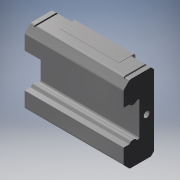
# Autodesk Inventor part: SRS12MSS Slider
Saved by Autodesk Inventor 2016 (Build 200138000, 138)
## iProperties
Category: PARTsolutions
Company: THK
Created: 2015-05-12
Part Number: SRS12MSS Slider
Catalog Web Link: www.cadenas.de
Description: Compact Type SRS-M Slider-
Vendor: THK
Document SubType Name: Modeling
Designer: PARTuser1
Manufacturer: THK
Mass: 57.6277 g
Surface Area: 35.5033 cm^2
Volume: 7.45507 cm^3
Density: 7.73 g/cm^3
Material: Steel, Alloy
Appearance: Semi-Polished
PSOL_IDENT_0: {$CADENAS_DATA\23d-libs\thk\linear_motion_systems\lm_guide\lm_caged_ball_roller\caged_ball\lm_guide_
PSOL_IDENT_1: srs\srs_m\srs_m_slider.prj},201 {VTYP=3D},{NB=SRS12MSS Slider},{LINA=SRS12MSS Slider},{NN=Compact Ty
PSOL_IDENT_2: pe SRS-M Slider},{DATE=07.01.2015 08:42:03},{GEOMDATE=07.01.2015 08:42:03},{VERSION=},{LINEID=130},{
PSOL_IDENT_3: LINESUBID=-1},{WBVAR=QZ,SO,GPJ}  {NB=SRS12MSS Slider},{LINA=SRS12MSS Slider},{KT=DUMMY},{MN=SRS12M},
PSOL_IDENT_4: {ND=3.000},{QZ=},{SO=SS},{SO1='SS','SS- With end seals, side seals','UU','UU- With end seals (on bot
PSOL_IDENT_5: h ends)','SSHH','SSHH- With end seals, side seals and LaCS'},{GPJ=},{M=13.00},{W=27.00},{K=11.00},{L=
PSOL_IDENT_6: 34.40},{L1=20.60},{LX=34.4},{B=20.00},{C=15.00},{S=3.00},{SL=3.200},{T=5.70},{N=3.00},{GPJ1='', 'Non
PSOL_IDENT_7: e'},{L4=0},{V=3.250},{M1=7.500},{X=3.500},{Y=2.000},{X1=0.500},{X2=26.800},{X3=4.800},{X4=3.000},{X5=
PSOL_IDENT_8: 3.000},{W1=12.000},{L3=5.400},{H3=2.000},{H=0.000},{QZ1='', 'No', 'QZ', 'Yes'},{UD1=21.000},{UD2=8.0
PSOL_IDENT_9: 00},{R=1.800},{VER=2},{VER2=2}
SUPPLIER: THK
ARTICLENO: SRS12MSS Slider
BOMINFO: SRS12MSS Slider
CREATOR: CADENAS GmbH
Title: SRS12MSS Slider
Author: Cadenas PARTsolutions
Autodesk Inventor part; units mm, degrees
sketch "Sketch_3" plane through (0, 0, 0) normal (1, 0, 0) x (0, 1, 0)
  line L0 (10.5, 13.5) -> (5.3, 13.5)
  line L1 (5.3, 13.5) -> (5.24, 13.4)
  line L2 (5.24, 13.4) -> (2.5142, 13.4)
  arc A0 (2.5142, 13.4) -> (1.8071, 13.1071) centre (2.5142, 12.4) ccw
  line L3 (1.8071, 13.1071) -> (0.2929, 11.5929)
  arc A1 (0.2929, 11.5929) -> (0, 10.8858) centre (1, 10.8858) ccw
  line L4 (0, 10.8858) -> (0, -10.8858)
  arc A2 (0, -10.8858) -> (0.2929, -11.5929) centre (1, -10.8858) ccw
  line L5 (0.2929, -11.5929) -> (1.8071, -13.1071)
  arc A3 (1.8071, -13.1071) -> (2.5142, -13.4) centre (2.5142, -12.4) ccw
  line L6 (2.5142, -13.4) -> (5.24, -13.4)
  line L7 (5.24, -13.4) -> (5.3, -13.5)
  line L8 (5.3, -13.5) -> (10.5, -13.5)
  line L9 (10.5, -13.5) -> (11, -13)
  line L10 (11, -13) -> (11, -6)
  line L11 (11, -6) -> (10.7713, -5.6188)
  arc A4 (10.7, -5.3615) -> (10.7713, -5.6188) centre (11.2, -5.3615) ccw
  line L12 (10.7, -5.3615) -> (10.7, 5.3615)
  arc A5 (10.7713, 5.6188) -> (10.7, 5.3615) centre (11.2, 5.3615) ccw
  line L13 (10.7713, 5.6188) -> (11, 6)
  line L14 (11, 6) -> (11, 13)
  line L15 (11, 13) -> (10.5, 13.5)
  constraints: 32 end point, 12 point on circle, 6 centre point
extrude "Extrusion1" add sketch "Sketch_3" along normal mid plane 20.6
sketch "Sketch_9" plane through (10.3, 0, 0) normal (1, 0, 0) x (0, 0, -1)
  arc A0 (-13.4, 2.5142) -> (-13.1071, 1.8071) centre (-12.4, 2.5142) ccw
  line L0 (-13.1071, 1.8071) -> (-11.5929, 0.2929)
  arc A1 (-11.5929, 0.2929) -> (-10.8858, 0) centre (-10.8858, 1) ccw
  line L1 (-10.8858, 0) -> (10.8858, 0)
  arc A2 (10.8858, 0) -> (11.5929, 0.2929) centre (10.8858, 1) ccw
  line L2 (11.5929, 0.2929) -> (13.1071, 1.8071)
  arc A3 (13.1071, 1.8071) -> (13.4, 2.5142) centre (12.4, 2.5142) ccw
  line L3 (13.4, 2.5142) -> (13.4, 9.5)
  line L4 (13.4, 9.5) -> (12.4, 10.5)
  line L5 (12.4, 10.5) -> (-12.4, 10.5)
  line L6 (-12.4, 10.5) -> (-13.4, 9.5)
  line L7 (-13.4, 9.5) -> (-13.4, 2.5142)
  constraints: 16 end point, 8 point on circle, 4 centre point
extrude "Extrusion2" add sketch "Sketch_9" along normal blind 6.9
sketch "Sketch_15" plane through (-10.3, 0, 0) normal (1, 0, 0) x (0, 0, -1)
  arc A0 (-13.4, 2.5142) -> (-13.1071, 1.8071) centre (-12.4, 2.5142) ccw
  line L0 (-13.1071, 1.8071) -> (-11.5929, 0.2929)
  arc A1 (-11.5929, 0.2929) -> (-10.8858, 0) centre (-10.8858, 1) ccw
  line L1 (-10.8858, 0) -> (10.8858, 0)
  arc A2 (10.8858, 0) -> (11.5929, 0.2929) centre (10.8858, 1) ccw
  line L2 (11.5929, 0.2929) -> (13.1071, 1.8071)
  arc A3 (13.1071, 1.8071) -> (13.4, 2.5142) centre (12.4, 2.5142) ccw
  line L3 (13.4, 2.5142) -> (13.4, 9.5)
  line L4 (13.4, 9.5) -> (12.4, 10.5)
  line L5 (12.4, 10.5) -> (-12.4, 10.5)
  line L6 (-12.4, 10.5) -> (-13.4, 9.5)
  line L7 (-13.4, 9.5) -> (-13.4, 2.5142)
  constraints: 16 end point, 8 point on circle, 4 centre point
extrude "Extrusion3" add sketch "Sketch_15" against normal blind 6.9
sketch "Sketch_40" plane through (0, 0, 0) normal (1, 0, 0) x (0, 1, 0)
  line L0 (-1.5, 6) -> (-2, 5.5)
  line L1 (-2, 5.5) -> (-2, -5.5)
  line L2 (-2, -5.5) -> (-1.5, -6)
  line L3 (-1.5, -6) -> (1.9874, -6)
  arc A0 (3.3, -5.2629) -> (1.9874, -6) centre (3.21, -6.64) ccw
  arc A1 (4.6126, -6) -> (3.3, -5.2629) centre (3.39, -6.64) ccw
  line L4 (4.6126, -6) -> (5.2, -6)
  line L5 (5.2, -6) -> (5.5, -5.7)
  line L6 (5.5, -5.7) -> (5.5, 5.7)
  line L7 (5.5, 5.7) -> (5.2, 6)
  line L8 (5.2, 6) -> (4.6126, 6)
  arc A2 (3.3, 5.2629) -> (4.6126, 6) centre (3.39, 6.64) ccw
  arc A3 (1.9874, 6) -> (3.3, 5.2629) centre (3.21, 6.64) ccw
  line L9 (1.9874, 6) -> (-1.5, 6)
  constraints: 20 end point, 8 point on circle, 4 centre point
extrude "Extrusion4" cut sketch "Sketch_40" along normal mid plane 34.4
sketch "Sketch5" plane through (-10.3, 11, 6) normal (0, 1, 0) x (1, 0, 0)
  point P0 (17.8, -4)
hole "Hole1" at (7.5, 11, 10) direction (0, -1, 0) diameter 2.459 depth 3.84 tip angle 120 countersink diameter 3 countersink angle 90 thread size "M3x0.5" class "6H" standard "ISO Metric profile"
pattern_linear "Rectangular Pattern1" count 2 spacing 20 along (0, 0, -1) count 2 spacing 15 along (-1, 0, 0) of "Hole1"
sketch "Sketch_38" plane through (0, 0, 0) normal (0, 0, 1) x (1, 0, 0)
  line L0 (15.2, 10.5) -> (15.7, 10)
  line L1 (15.7, 10) -> (15.7, 10.5)
  line L2 (15.7, 10.5) -> (15.2, 10.5)
  constraints: 6 end point
extrude "Extrusion5" cut sketch "Sketch_38" along normal mid plane 26.8
sketch "Sketch_39" plane through (0, 0, 0) normal (0, 0, 1) x (1, 0, 0)
  line L0 (-15.7, 10.5) -> (-15.7, 10)
  line L1 (-15.7, 10) -> (-15.2, 10.5)
  line L2 (-15.2, 10.5) -> (-15.7, 10.5)
  constraints: 6 end point
extrude "Extrusion6" cut sketch "Sketch_39" along normal mid plane 26.8
sketch "Sketch_21" plane through (0, 0, 0) normal (0, 1, 0) x (-1, 0, 0)
  line L0 (15.7, -13.4) -> (15.7, -12.9)
  line L1 (15.7, -12.9) -> (15.2, -13.4)
  line L2 (15.2, -13.4) -> (15.7, -13.4)
  constraints: 6 end point
extrude "Extrusion7" cut sketch "Sketch_21" along normal blind 11
sketch "Sketch_22" plane through (0, 0, 0) normal (0, 1, 0) x (-1, 0, 0)
  line L0 (-15.2, -13.4) -> (-15.7, -12.9)
  line L1 (-15.7, -12.9) -> (-15.7, -13.4)
  line L2 (-15.7, -13.4) -> (-15.2, -13.4)
  constraints: 6 end point
extrude "Extrusion8" cut sketch "Sketch_22" along normal blind 11
sketch "Sketch_23" plane through (0, 0, 0) normal (0, 1, 0) x (-1, 0, 0)
  line L0 (-15.2, 13.4) -> (-15.7, 13.4)
  line L1 (-15.7, 13.4) -> (-15.7, 12.9)
  line L2 (-15.7, 12.9) -> (-15.2, 13.4)
  constraints: 6 end point
extrude "Extrusion9" cut sketch "Sketch_23" along normal blind 11
sketch "Sketch_24" plane through (0, 0, 0) normal (0, 1, 0) x (-1, 0, 0)
  line L0 (15.7, 13.4) -> (15.2, 13.4)
  line L1 (15.2, 13.4) -> (15.7, 12.9)
  line L2 (15.7, 12.9) -> (15.7, 13.4)
  constraints: 6 end point
extrude "Extrusion10" cut sketch "Sketch_24" along normal blind 11
sketch "Sketch12" plane through (17.2, 0, 0) normal (1, 0, 0) x (0, 0, -1)
  point P0 (0, 8)
hole "Hole2" at (17.2, 8, 0) direction (-1, 0, 0) diameter 2 depth 3.5
sketch "Sketch_32" plane through (0, 0, 0) normal (0, 0, 1) x (1, 0, 0)
  line L0 (-13.7, 8) -> (-17.2, 8)
  line L1 (-17.2, 8) -> (-17.2, 9)
  line L2 (-17.2, 9) -> (-13.7, 9)
  line L3 (-13.7, 9) -> (-13.7, 8)
  line L4 (-13.7, 8) -> (-17.2, 8)
  constraints: 10 end point
revolve "Revolution1" cut sketch "Sketch_32" angle 360 about axis through (-13.7, 8, 0) along (1, 0, 0)
ref_plane "4track_XY" through (0, 0, 0) normal (1, 0, 0) x (0, 0, -1)
ref_plane "4track_YZ" through (0, 0, 0) normal (0, 0, -1) x (0, 1, 0)
ref_plane "4track_ZX" through (0, 0, 0) normal (0, 1, 0) x (1, 0, 0)
body "Solid1"
